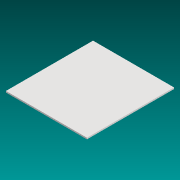
# Autodesk Inventor part: 导轨
Saved by Autodesk Inventor 2021 (Build 250183000, 183)
## iProperties
Created: 2025-04-17
Part Number: 导轨
Material: 常规
Document SubType Name: Modeling
Designer: 86155
Density: 1 g/cm^3
Appearance: 默认
Author: 86155
Autodesk Inventor part; units mm, degrees
ref_plane "YZ Plane" through (0, 0, 0) normal (1, 0, 0) x (0, 1, 0)
ref_plane "XZ Plane" through (0, 0, 0) normal (0, 1, 0) x (-1, 0, 0)
ref_plane "XY Plane" through (0, 0, 0) normal (0, 0, 1) x (1, 0, 0)
sketch "草图1" plane through (0, 0, 0) normal (0, 1, 0) x (-1, 0, 0)
  line L0 (41.3476, 0) -> (-48.6524, 0)
  line L1 (-48.6524, 0) -> (-48.6524, -96.7534)
  line L2 (-48.6524, -96.7534) -> (41.3476, -96.7534)
  line L3 (41.3476, -96.7534) -> (41.3476, 0)
  point P0 (0, 0)
  dimension "d2" = 90
  constraints: 8 end point, 2 parallel, 1 horizontal, 1 perpendicular
  measures "d2" distance between parallel lines of L1 L3
extrude "拉伸1" add sketch "草图1" along normal blind 1
